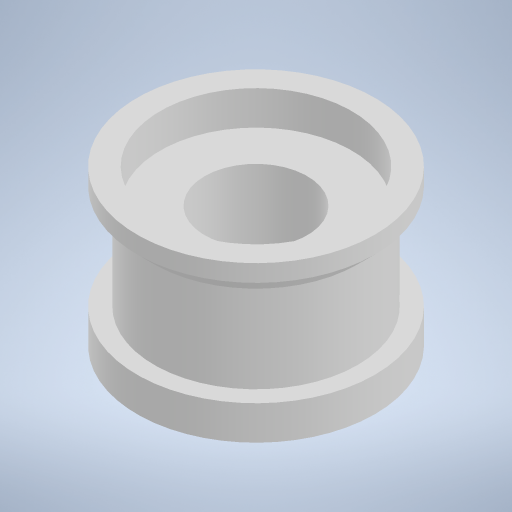
# Autodesk Inventor part: SolarPlugAdapter
Saved by Autodesk Inventor 2024 (Build 280153000, 153)
## iProperties
Created: 2025-03-02
Part Number: SolarPlugAdapter
Material: Generisch
Document SubType Name: Modeling
Designer: maxho
Density: 1 g/cm^3
Appearance: Vorgabe
Author: maxho
## iProperties of the stored document MemberDocs/xH1vu03xxKsvxvkjl1qcvhdq3La
Created: 2025-03-02
Part Number: SolarPlugAdapter
Material: Generisch
Document SubType Name: Modeling
Designer: maxho
Density: 1 g/cm^3
Appearance: Vorgabe
Author: maxho
## iProperties of the stored document SolarPlugAdapter_3D-Druck.ipt
Created: 2025-03-02
Part Number: SolarPlugAdapter_3D-Druck
Material: Generisch
Document SubType Name: Modeling
Designer: maxho
Density: 1 g/cm^3
Appearance: Vorgabe
Author: maxho
Autodesk Inventor part; units mm, degrees
ref_plane "YZ Plane" through (0, 0, 0) normal (1, 0, 0) x (0, 1, 0)
ref_plane "XZ Plane" through (0, 0, 0) normal (0, 1, 0) x (-1, 0, 0)
ref_plane "XY Plane" through (0, 0, 0) normal (0, 0, 1) x (1, 0, 0)
sketch "Skizze1" plane through (0, 0, 0) normal (0, 0, 1) x (1, 0, 0)
  circle A0 centre (0, 0) radius 5.95
  dimension "d0" = 11.9
  constraints: 1 centre point, 1 coincident
  measures "d0" diameter of A0
extrude "Extrusion1" add sketch "Skizze1" along normal blind 2.55
sketch "Skizze2" plane through (0, 0, 2.55) normal (0, 0, 1) x (1, 0, 0)
  circle A0 centre (0, 0) radius 6.95
  circle A1 centre (0, 0) radius 5.95 projected
  dimension "d5" = 1
  constraints: 1 centre point, 1 coincident
  measures "d5" radial gap between concentric circles of A0 A1
extrude "Extrusion2" add sketch "Skizze2" along normal blind 2 contours A0 | A1
mirror "Spiegeln1" about plane through (0, 0, 0) normal (0, 0, -1) of "Extrusion2", "Extrusion1"
sketch "Skizze3" plane through (0, 0, 4.55) normal (0, 0, 1) x (1, 0, 0)
  point P0 (0, 0)
  point P1 (0, 0)
  constraints: 1 coincident
hole "Bohrung1" at (0, 0, 4.55) direction (0, 0, -1) diameter 6 end through all counterbore diameter 11.2 counterbore depth 2
chamfer "Fasen1" distance 1 angle 45 1 edges at (-6.95, 0, 2.55)
